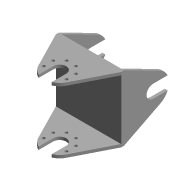
# Autodesk Inventor part: Ankle
Saved by Autodesk Inventor 2011 (Build 150239000, 239)
## iProperties
Created: 2010-11-21
Part Number: Ankle
Document SubType Name: Modeling
Designer: Milton
Density: 1 g/cm^3
Mass: 10.0039 g
Surface Area: 111.469 cm^2
Volume: 10.0039 cm^3
Author: Milton
Autodesk Inventor part; units mm, degrees
ref_plane "YZ Plane" through (0, 0, 0) normal (1, 0, 0) x (0, 1, 0)
ref_plane "XZ Plane" through (0, 0, 0) normal (0, 1, 0) x (-1, 0, 0)
ref_plane "XY Plane" through (0, 0, 0) normal (0, 0, 1) x (1, 0, 0)
sketch "Sketch1" plane through (0, 0, 0) normal (0, 0, 1) x (1, 0, 0)
  line L0 (9.7751, 75.6011) -> (11.7751, 75.6011)
  line L1 (52.7751, 75.6011) -> (54.7751, 75.6011)
  arc A0 (22.5579, 17.6142) -> (42.1677, 17.6615) centre (32.3508, 22.6241) ccw
  line L2 (9.7751, 42.6011) -> (54.7751, 42.6011)
  line L3 (11.7751, 44.6011) -> (52.7751, 44.6011)
  line L4 (11.7751, 75.6011) -> (11.7751, 44.6011)
  line L5 (9.7751, 75.6011) -> (9.7751, 42.6011)
  line L6 (52.7751, 75.6011) -> (52.7751, 44.6011)
  line L7 (54.7751, 75.6011) -> (54.7751, 42.6011)
  line L8 (54.7751, 42.6011) -> (42.1677, 17.6615)
  line L9 (9.7751, 42.6011) -> (22.5579, 17.6142)
  circle A1 centre (32.3508, 22.6241) radius 4.5
  point P0 (0, 0)
  dimension "d15" = 9
  constraints: 20 end point, 2 centre point, 2 point on circle, 1 coincident
  measures "d15" diameter of A1
extrude "Extrusion1" add sketch "Sketch1" against normal blind 45
sketch "Sketch2" plane through (54.7751, 42.6011, 0) normal (1, 0, 0) x (0, 0, -1)
  circle A0 centre (22.5, 22) radius 11
  line L0 (0, 0) -> (0, 2)
  line L1 (0, 33) -> (0, 0) projected
  line L2 (45, 0) -> (45, 2)
  line L3 (45, 33) -> (45, 0) projected
  line L4 (45, 2) -> (32.3068, 26.9826)
  line L5 (0, 2) -> (12.6932, 26.9826)
  line L6 (0, 2) -> (0, 38)
  line L7 (0, 38) -> (45, 38)
  line L8 (45, 38) -> (45, 2)
  circle A1 centre (22.5, 22) radius 4.5
  line L9 (0, 0) -> (45, 0)
  line L10 (45, -24.9396) -> (45, 0) projected
  point P0 (0, -42.6011)
  dimension "d2" = 22
  dimension "d16" = 9
  constraints: 16 end point, 2 centre point, 2 point on circle, 2 point on line, 2 tangent, 1 coincident, 1 perpendicular
  measures "d2" diameter of A0
  measures "d16" diameter of A1
extrude "Extrusion2" cut sketch "Sketch2" against normal blind 45 contours A0 L5 L1 L6 L7 L8 L3 L4 | A1
sketch "Sketch3" plane through (54.7751, 42.6011, 0) normal (1, 0, 0) x (0, 0, -1)
  line L0 (0, 0) -> (45, 0) projected
  line L1 (43, 0) -> (2, 0)
  line L2 (2, 0) -> (2, -33)
  line L3 (2, -33) -> (43, -33)
  line L4 (43, -33) -> (43, 0)
  line L5 (45, -24.9396) -> (45, 0) projected
  point P0 (0, -42.6011)
  dimension "d9" = 41
  dimension "d10" = 2
  constraints: 8 end point, 2 parallel, 1 horizontal, 1 perpendicular, 1 point on line
  measures "d9" distance of L3.end L2.end
  measures "d10" distance between parallel lines of L5 L4
extrude "Extrusion3" cut sketch "Sketch3" against normal blind 45
sketch "Sketch5" plane through (0, 0, 0) normal (0, 0, 1) x (1, 0, 0)
  line L0 (9.7751, 42.6011) -> (22.5579, 17.6142) projected
  arc A0 (22.5579, 17.6142) -> (42.1677, 17.6615) centre (32.3508, 22.6241) ccw projected
  line L1 (42.1677, 17.6615) -> (54.7751, 42.6011) projected
  line L2 (52.7751, 44.6011) -> (11.7751, 44.6011) projected
  circle A1 centre (32.3508, 22.6241) radius 4.5 projected
  line L3 (27.8508, 22.6241) -> (27.8508, 12.5867)
  line L4 (36.8508, 22.6241) -> (36.8508, 12.5867)
  arc A2 (36.8508, 22.6241) -> (27.8508, 22.6241) centre (32.3508, 22.6241) ccw
  arc A3 (27.8508, 12.5867) -> (36.8508, 12.5867) centre (32.3508, 22.6241) ccw
  point P0 (0, 0)
  constraints: 8 point on circle, 6 end point, 2 centre point, 2 coincident, 2 concentric, 2 tangent, 1 parallel, 1 perpendicular
extrude "Extrusion4" cut sketch "Sketch5" against normal through all
sketch "Sketch6" plane through (54.7751, 42.6011, 0) normal (1, 0, 0) x (0, 0, -1)
  arc A0 (32.3068, 26.9826) -> (12.6932, 26.9826) centre (22.5, 22) ccw projected
  arc A1 (18, 22) -> (27, 22) centre (22.5, 22) ccw
  line L0 (18, 22) -> (18, 34.9118)
  line L1 (27, 22) -> (27, 34.9118)
  line L2 (27, 34.9118) -> (18, 34.9118)
  point P0 (0, -42.6011)
  dimension "d19" = 9
  constraints: 6 end point, 2 point on circle, 2 tangent, 1 centre point, 1 coincident, 1 parallel, 1 perpendicular
  measures "d19" diameter of A1
extrude "Extrusion5" cut sketch "Sketch6" against normal through all
sketch "Sketch7" plane through (0, 0, -45) normal (0, 0, -1) x (-1, 0, 0)
  arc A0 (-27.8508, 12.5867) -> (-22.5579, 17.6142) centre (-32.3508, 22.6241) ccw projected
  circle A1 centre (-24.4978, 25.8769) radius 1
  point P0 (0, 0)
  dimension "d22" = 2
  dimension "d23" = 8.5
  constraints: 1 centre point
  measures "d22" diameter of A1
  measures "d23" distance of A1.centre A0.centre
extrude "Extrusion6" cut sketch "Sketch7" against normal through all
pattern_circular "Circular Pattern1" count 8 over 360 about axis through (32.3508, 22.6241, 0) along (0, 0, -1) of "Extrusion6"
sketch "Sketch8" plane through (9.7751, 42.6011, 0) normal (-1, 0, 0) x (0, 0, 1)
  arc A0 (-27, 22) -> (-18, 22) centre (-22.5, 22) ccw projected
  line L0 (-22.5, 22) -> (-14.647, 25.2528)
  line L1 (-22.5, 22) -> (-14, 22) construction
  circle A1 centre (-14.647, 25.2528) radius 1
  point P0 (0, -42.6011)
  dimension "d29" = 8.5
  dimension "d30" = 22.5
  dimension "d31" = 2
  constraints: 4 end point, 1 centre point, 1 coincident, 1 equal length, 1 horizontal
  measures "d29" distance of L0.start L0.end
  measures "d30" angle of L1 L0
  measures "d31" diameter of A1
extrude "Extrusion7" cut sketch "Sketch8" against normal through all
pattern_circular "Circular Pattern2" count 8 over 360 about axis through (54.7751, 64.6011, -22.5) along (-1, 0, 0) of "Extrusion7"
body "Solid1"
